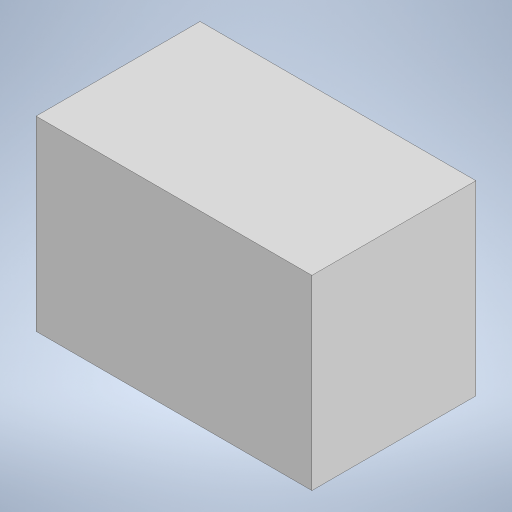
# Autodesk Inventor part: switch
Saved by Autodesk Inventor 2024 (Build 280153000, 153)
## iProperties
Created: 2023-12-14
Part Number: switch
Material: Ogólny
Document SubType Name: Modeling
Designer: pient
Density: 1 g/cm^3
Appearance: Domyślna
Author: pient
Autodesk Inventor part; units mm, degrees
ref_plane "YZ Plane" through (0, 0, 0) normal (1, 0, 0) x (0, 1, 0)
ref_plane "XZ Plane" through (0, 0, 0) normal (0, 1, 0) x (-1, 0, 0)
ref_plane "XY Plane" through (0, 0, 0) normal (0, 0, 1) x (1, 0, 0)
sketch "Szkic1" plane through (0, 0, 0) normal (0, 0, 1) x (1, 0, 0)
  line L0 (-9.25, 6.25) -> (9.25, 6.25)
  line L1 (9.25, 6.25) -> (9.25, -6.25)
  line L2 (9.25, -6.25) -> (-9.25, -6.25)
  line L3 (-9.25, -6.25) -> (-9.25, 6.25)
  point P0 (0, 0)
  dimension "d0" = 18.5
  dimension "d1" = 12.5
  dimension "d2" = 9.25
  dimension "d3" = 6.25
  constraints: 8 end point, 2 parallel, 1 horizontal, 1 perpendicular
  measures "d0" distance of L1.end L2.end
  measures "d1" distance of L0.end L1.end
  measures "d2" horizontal distance of L1.end point (0, 0)
  measures "d3" vertical distance of L1.end point (0, 0)
extrude "Wyciągnięcie proste1" add sketch "Szkic1" along normal blind 11
